sliderrailfader (Autodesk Fusion 360 design; units mm, degrees)
Autodesk Fusion 360 part; units mm, degrees
sketch "Sketch1" plane through (0, 0, 0) normal (0, 1, 0) x (1, 0, 0)
  line L0 (0, 0) -> (53, 0)
  line L1 (53, 0) -> (53, -7)
  line L2 (53, -7) -> (0, -7)
  line L3 (0, -7) -> (0, 0)
  line L4 (0, -3.5) -> (53, -3.5)
  line L5 (0, -3.5) -> (0, -11.5)
  line L6 (0, -3.5) -> (0, 4.5)
  line L7 (0, 4.5) -> (-10, 4.5)
  line L8 (-10, 4.5) -> (-10, -11.5)
  line L9 (-10, -11.5) -> (0, -11.5)
  line L10 (0, -11.5) -> (0, 4.5)
  line L11 (53, -3.5) -> (53, 4.5)
  line L12 (53, -3.5) -> (53, -11.5)
  line L13 (53, 4.5) -> (63, 4.5)
  line L14 (63, 4.5) -> (63, -11.5)
  line L15 (63, -11.5) -> (53, -11.5)
  line L16 (53, -11.5) -> (53, 4.5)
  line L17 (-10, 4.5) -> (63, 4.5)
  line L18 (63, 4.5) -> (63, -11.5)
  line L19 (63, -11.5) -> (-10, -11.5)
  line L20 (-10, -11.5) -> (-10, 4.5)
  line L21 (0, -3.5) -> (4, -3.5)
  circle A0 centre (4, -3.5) radius 0.5
  line L22 (4, -3.5) -> (19, -3.5)
  line L23 (19, -3.5) -> (34, -3.5)
  line L24 (34, -3.5) -> (49, -3.5)
  circle A1 centre (19, -3.5) radius 0.5
  circle A2 centre (34, -3.5) radius 0.5
  circle A3 centre (49, -3.5) radius 0.5
  line L25 (-10, -3.5) -> (-10, -12.5)
  line L26 (-10, -3.5) -> (-10, 5.5)
  line L27 (63, -3.5) -> (63, 5.5)
  line L28 (63, -3.5) -> (63, -12.5)
  line L29 (-10, 5.5) -> (63, 5.5)
  line L30 (63, 5.5) -> (63, -12.5)
  line L31 (63, -12.5) -> (-10, -12.5)
  line L32 (-10, -12.5) -> (-10, 5.5)
  line L33 (-10, -12.5) -> (63, -12.5)
  line L34 (63, -12.5) -> (63, -17.5)
  line L35 (63, -17.5) -> (-10, -17.5)
  line L36 (-10, -17.5) -> (-10, -12.5)
  line L37 (-10, 5.5) -> (63, 5.5)
  line L38 (63, 5.5) -> (63, 10.5)
  line L39 (63, 10.5) -> (-10, 10.5)
  line L40 (-10, 10.5) -> (-10, 5.5)
  line L41 (0, -3.5) -> (-5, -3.5)
  line L42 (53, -3.5) -> (58, -3.5)
  circle A4 centre (-5, -3.5) radius 1.5
  circle A5 centre (58, -3.5) radius 1.5
  dimension "d1" = 7
  dimension "d2" = 53
  dimension "d3" = 8
  dimension "d4" = 8
  dimension "d5" = 10
  dimension "d6" = 8
  dimension "d7" = 8
  dimension "d8" = 10
  dimension "d9" = 4
  dimension "d10" = 1
  dimension "d11" = 15
  dimension "d12" = 15
  dimension "d13" = 15
  dimension "d14" = 1
  dimension "d15" = 1
  dimension "d16" = 1
  dimension "d27" = 9
  dimension "d28" = 9
  dimension "d29" = 9
  dimension "d30" = 9
  dimension "d31" = 5
  dimension "d32" = 5
  dimension "d41" = 5
  dimension "d42" = 5
  dimension "d43" = 3
  dimension "d44" = 3
  constraint horizontal L0
  constraint vertical L1
  constraint horizontal L2
  constraint vertical L3
  constraint coincident L0.start L3.end
  constraint midpoint L3 L4.start
  constraint midpoint L1 L4.end
  constraint perpendicular L2 L5
  constraint perpendicular L4 L6
  constraint horizontal L7
  constraint vertical L8
  constraint horizontal L9
  constraint vertical L10
  constraint perpendicular L0 L11
  constraint perpendicular L2 L12
  constraint horizontal L13
  constraint vertical L14
  constraint horizontal L15
  constraint vertical L16
  constraint horizontal L17
  constraint vertical L18
  constraint horizontal L19
  constraint vertical L20
  constraint perpendicular L6 L21
  constraint coincident L21.end A0.centre
  constraint parallel L4 L22
  constraint parallel L4 L23
  constraint parallel L4 L24
  constraint coincident L22.end L23.start
  constraint coincident L23.end L24.start
  constraint coincident L24.end A3.centre
  constraint midpoint L8 L25.start
  constraint perpendicular L19 L25
  constraint perpendicular L7 L26
  constraint midpoint L14 L27.start
  constraint parallel L14 L27
  constraint perpendicular L15 L28
  constraint horizontal L29
  constraint vertical L30
  constraint horizontal L31
  constraint vertical L32
  constraint horizontal L33
  constraint vertical L34
  constraint horizontal L35
  constraint vertical L36
  constraint horizontal L37
  constraint vertical L38
  constraint horizontal L39
  constraint vertical L40
  constraint perpendicular L20 L41
  constraint perpendicular L1 L42
  constraint coincident L41.end A4.centre
  constraint coincident L42.end A5.centre
  measures "d1" distance of L0.start L2.end
  measures "d2" distance of L0.start L0.end
  measures "d3" distance of L4.start L5.end
  measures "d4" distance of L4.start L6.end
  measures "d5" distance of L6.end L7.end
  measures "d6" distance of L4.end L11.end
  measures "d7" distance of L4.end L12.end
  measures "d8" distance of L11.end L13.end
  measures "d9" distance of L4.start L21.end
  measures "d10" diameter of A0
  measures "d11" distance of L21.end L22.end
  measures "d12" distance of L22.end L23.end
  measures "d13" distance of L23.end L24.end
  measures "d14" diameter of A1
  measures "d15" diameter of A2
  measures "d16" diameter of A3
  measures "d27" distance of L25.start L25.end
  measures "d28" distance of L25.start L26.end
  measures "d29" distance of L27.start L27.end
  measures "d30" distance of L27.start L28.end
  measures "d31" distance of L25.end L35.end
  measures "d32" distance of L26.end L39.end
  measures "d41" distance of L4.start L41.end
  measures "d42" distance of L4.end L42.end
  measures "d43" diameter of A4
  measures "d44" diameter of A5
extrude "Extrude1" add sketch "Sketch1" along normal blind 1 contours L0 L6 L10 L11 L16 L17 | L2 L5 L10 L12 L16 L19 makes body 1 at (17.6667, 0, -3) makes body 2 at (17.6667, 0, 8.5)
extrude "Extrude2" add sketch "Sketch1" along normal blind 9 contours L3 L5 L6 L7 L8 L9 L10 L17 L19 L20 L25 L26 L32 | L1 L11 L12 L13 L14 L15 L16 L17 L18 L19 L27 L28 L30 | A4 | A5 bodies 1 2
extrude "Extrude3" cut 2 faces at (-6.6667, 9, 6.1667) (56.3333, 9, 6.1667) along direction (0, -1, 0) blind 1 on bodies 1 bodies 1
extrude "Extrude4" add 1 faces at (-6.6667, 3, 11.5) along direction (0, 0, 1) blind 1 on bodies 1 bodies 1
extrude "Extrude5" add 1 faces at (-6.6667, 3, -4.5) along direction (0, 0, -1) blind 1 on bodies 1 bodies 1
extrude "Extrude6" add sketch "Sketch1" along normal blind 8 contours L29 L37 L38 L39 L40 | L31 L33 L34 L35 L36 bodies 1
extrude "Extrude7" add sketch "Sketch1" against normal blind 5 contours L0 L6 L10 L11 L16 L17 | L0 L1 L3 L4 L6 L10 L11 L16 L21 A0 L22 L23 L24 A1 A2 A3 | L3 L5 L6 L7 L8 L9 L10 L17 L19 L20 L25 L26 L32 | L1 L11 L12 L13 L14 L15 L16 L17 L18 L19 L27 L28 L30 | L1 L2 L3 L4 L5 L10 L12 L16 L21 A0 L22 L23 L24 A1 A2 A3 | L7 L13 L17 L26 L27 L29 L30 L32 L37 | L2 L5 L10 L12 L16 L19 | L9 L15 L19 L25 L28 L30 L31 L32 L33 | L29 L37 L38 L39 L40 | L31 L33 L34 L35 L36 | A4 | A5 bodies 1
chamfer "Chamfer1" distance 1.5 angle 45 4 edges at (48.5338, 0, 3.3192) (33.5338, 0, 3.3192) (18.5338, 0, 3.3192) (3.5338, 0, 3.3192) on bodies 1
chamfer "Chamfer2" distance 0.5 angle 45 2 edges at (26.5, 1, 7) (26.5, 1, 0) on bodies 1
chamfer "Chamfer3" distance 2 angle 45 4 edges at (26.5, 8, -5.5) (53, 8, 3.5) (26.5, 8, 12.5) (0, 8, 3.5) on bodies 1
chamfer "Chamfer4" distance 2 angle 45 4 edges at (26.5, 8, -10.5) (63, 8, 3.5) (26.5, 8, 17.5) (-10, 8, 3.5) on bodies 1
extrude "Extrude8" cut sketch "Sketch1" along normal mid plane 40 contours A4 | A5 bodies 1
chamfer "Chamfer5" distance 2 angle 45 2 edges at (-6.3985, 8, 2.9576) (56.6015, 8, 2.9576) on bodies 1
